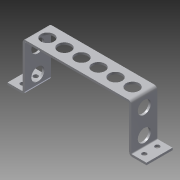
# Autodesk Inventor part: M - Lower Rail Connector Bracket 1
Saved by Autodesk Inventor 2013 (Build 170138000, 138)
## iProperties
Created: 2013-02-17
Part Number: M - Lower Rail Connector Bracket 1
Material: Aluminum 6061
Document SubType Name: Sheet Metal
Designer: Moses
Density: 2.71 g/cm^3
Sheet Metal Rule: Default
Mass: 82.9622 g
Surface Area: 238.016 cm^2
Volume: 30.6134 cm^3
Author: Moses
Autodesk Inventor part; units mm, degrees
ref_plane "YZ Plane" through (0, 0, 0) normal (1, 0, 0) x (0, 1, 0)
ref_plane "XZ Plane" through (0, 0, 0) normal (0, 1, 0) x (-1, 0, 0)
ref_plane "XY Plane" through (0, 0, 0) normal (0, 0, 1) x (1, 0, 0)
sketch "Sketch1" plane through (0, 0, 0) normal (0, 1, 0) x (-1, 0, 0)
  line L0 (0, 0) -> (0, 38.1)
  line L1 (0, 38.1) -> (25.4, 38.1)
  line L2 (25.4, 38.1) -> (25.4, 0)
  line L3 (25.4, 0) -> (0, 0)
  line L4 (12.7, 38.1) -> (12.7, 0) construction
  circle A0 centre (12.7, 28.575) radius 3.3782
  circle A1 centre (12.7, 9.525) radius 3.3782
  dimension "d0" = 38.1
  dimension "d1" = 25.4
  dimension "d2" = 6.7564
  dimension "d3" = 19.05
  dimension "d4" = 9.525
  measures "d0" distance of L0.start L0.end
  measures "d1" distance of L0.end L1.end
  measures "d2" diameter of A0
  measures "d3" distance of A1.centre A0.centre
  measures "d4" distance from line of L1 A0.centre
extrude "Plate1" add sketch "Sketch1" along normal blind 3.175
sketch "Sketch2" plane through (-22.225, 0, 38.1) normal (-1, 0, 0) x (0, -1, 0)
  line L0 (0, -38.1) -> (0, 0)
  line L1 (0, 0) -> (-69.85, 0)
  line L2 (-69.85, 0) -> (-69.85, -38.1)
  line L3 (-69.85, -38.1) -> (0, -38.1)
  constraints: 6 end point, 1 horizontal, 1 perpendicular, 1 vertical
edge flange "Flange1" height 69.85 angle 90 thickness 3.175 bend radius 1.27 thickness toward (-1, 0, 0) relief tear relief width 3.175 relief depth 1.5875 edges at (-25.4, 3.175, 19.05) wall of the first edge with corners at (-22.225, 0, 0) (-22.225, 0, 38.1) (-22.225, 69.85, 38.1) (-22.225, 69.85, 0)
bend "Bend1"
corner "Corner1"
sketch "Sketch3" plane through (-22.225, 66.675, 0) normal (0, 1, 0) x (-1, 0, 0)
  line L0 (0, 38.1) -> (0, 0)
  line L1 (0, 0) -> (158.75, 0)
  line L2 (158.75, 0) -> (158.75, 38.1)
  line L3 (158.75, 38.1) -> (0, 38.1)
  constraints: 6 end point, 1 horizontal, 1 perpendicular, 1 vertical
edge flange "Flange2" height 158.75 angle 90 thickness 3.175 bend radius 1.27 thickness toward (0, 1, 0) relief tear relief width 3.175 relief depth 1.5875 edges at (-25.4, 69.85, 19.05) wall of the first edge with corners at (-22.225, 66.675, 38.1) (-22.225, 66.675, 0) (-180.975, 66.675, 0) (-180.975, 66.675, 38.1)
bend "Bend2"
corner "Corner2"
sketch "Sketch4" plane through (-177.8, 69.85, 0) normal (-1, 0, 0) x (0, -1, 0)
  line L0 (0, 38.1) -> (0, 0)
  line L1 (0, 0) -> (69.85, 0)
  line L2 (69.85, 0) -> (69.85, 38.1)
  line L3 (69.85, 38.1) -> (0, 38.1)
  constraints: 6 end point, 1 horizontal, 1 perpendicular, 1 vertical
edge flange "Flange3" height 69.85 angle 90 thickness 3.175 bend radius 1.27 thickness toward (-1, 0, 0) relief tear relief width 3.175 relief depth 1.5875 edges at (-180.975, 66.675, 19.05) wall of the first edge with corners at (-177.8, 69.85, 38.1) (-177.8, 69.85, 0) (-177.8, 0, 0) (-177.8, 0, 38.1)
bend "Bend3"
corner "Corner3"
sketch "Sketch5" plane through (-177.8, 3.175, 38.1) normal (0, -1, 0) x (1, 0, 0)
  line L0 (0, -38.1) -> (0, 0)
  line L1 (0, 0) -> (-25.4, 0)
  line L2 (-25.4, 0) -> (-25.4, -38.1)
  line L3 (-25.4, -38.1) -> (0, -38.1)
  constraints: 6 end point, 1 horizontal, 1 perpendicular, 1 vertical
edge flange "Flange4" height 25.4 angle 90 thickness 3.175 bend radius 1.27 thickness toward (0, -1, 0) relief tear relief width 3.175 relief depth 1.5875 edges at (-180.975, 0, 19.05) wall of the first edge with corners at (-177.8, 3.175, 0) (-177.8, 3.175, 38.1) (-203.2, 3.175, 38.1) (-203.2, 3.175, 0)
bend "Bend4"
corner "Corner4"
sketch "Sketch6" plane through (-203.2, 0, 0) normal (0, -1, 0) x (1, 0, 0)
  line L0 (0, 38.1) -> (20.955, 38.1) projected
  line L1 (0, 0) -> (0, 38.1) projected
  line L2 (20.955, 0) -> (0, 0) projected
  line L3 (12.7, 38.1) -> (12.7, 0) construction
  circle A0 centre (12.7, 28.575) radius 3.3782
  circle A1 centre (12.7, 9.525) radius 3.3782
  point P0 (203.2, 0)
  dimension "d46" = 12.7
  dimension "d47" = 6.7564
  dimension "d48" = 19.05
  dimension "d49" = 9.525
  constraints: 4 point on line, 2 centre point, 2 end point, 1 equal radius, 1 perpendicular
  measures "d46" distance between parallel lines of L3 L1
  measures "d47" diameter of A0
  measures "d48" distance of A1.centre A0.centre
  measures "d49" distance from line of L0 A0.centre
extrude "Cut1" cut sketch "Sketch6" against normal blind 3.175
sketch "Sketch7" plane through (-26.67, 69.85, 38.1) normal (0, 1, 0) x (1, 0, 0)
  line L0 (-149.86, 38.1) -> (-149.86, 0) projected
  line L1 (0, 0) -> (0, 38.1) projected
  circle A0 centre (-137.16, 19.05) radius 9.525
  line L2 (-149.86, 19.05) -> (0, 19.05) construction
  circle A1 centre (-112.268, 19.05) radius 9.525
  circle A2 centre (-87.376, 19.05) radius 9.525
  circle A3 centre (-62.484, 19.05) radius 9.525
  circle A4 centre (-37.592, 19.05) radius 9.525
  circle A5 centre (-12.7, 19.05) radius 9.525
  point P0 (26.67, 38.1)
  dimension "d52" = 149.86
  dimension "d53" = 12.7
  dimension "d56" = 24.892
  dimension "d61" = 19.05
  constraints: 6 centre point, 2 end point, 2 midpoint, 1 horizontal, 1 point on line, 10 other
  measures "d52" distance of L0.start L1.end
  measures "d53" distance from line of A0.centre L0
  measures "d56" distance of A0.centre A1.centre
  measures "d61" diameter of A0
extrude "Cut2" cut sketch "Sketch7" against normal blind 3.175
sketch "Sketch8" plane through (-180.975, 65.405, 0) normal (-1, 0, 0) x (0, 0, 1)
  line L0 (0, -60.96) -> (38.1, -60.96) projected
  line L1 (38.1, 0) -> (0, 0) projected
  line L2 (19.05, 0) -> (19.05, -60.96) construction
  circle A0 centre (19.05, -12.7) radius 9.525
  circle A1 centre (19.05, -48.26) radius 9.525
  point P0 (0, -65.405)
  dimension "d64" = 19.05
  dimension "d66" = 12.7
  dimension "d67" = 12.7
  constraints: 2 centre point, 2 end point, 2 midpoint, 2 point on line, 1 equal radius
  measures "d64" diameter of A0
  measures "d66" distance from line of L1 A0.centre
  measures "d67" distance from line of L0 A1.centre
extrude "Cut3" cut sketch "Sketch8" against normal blind 5080
equation "\"d50\" = Thickness"
equation "\"d56\" = -0.4 * d53 + 0.2 * d52"
equation "\"d62\" = Thickness"
equation "\"d6\" = BendReliefWidth"
equation "\"d7\" = BendReliefDepth"
equation "\"d8\" = MinimumRemnant"
equation "\"d9\" = BendRadius"
equation "\"d13\" = CornerReliefSize"
equation "\"d14\" = GapSize"
equation "\"d15\" = JacobiRadiusSize"
equation "\"d16\" = BendReliefWidth"
equation "\"d17\" = BendReliefDepth"
equation "\"d18\" = MinimumRemnant"
equation "\"d19\" = BendRadius"
equation "\"d23\" = CornerReliefSize"
equation "\"d24\" = GapSize"
equation "\"d25\" = JacobiRadiusSize"
equation "\"d26\" = BendReliefWidth"
equation "\"d27\" = BendReliefDepth"
equation "\"d28\" = MinimumRemnant"
equation "\"d29\" = BendRadius"
equation "\"d33\" = CornerReliefSize"
equation "\"d34\" = GapSize"
equation "\"d35\" = JacobiRadiusSize"
equation "\"d36\" = BendReliefWidth"
equation "\"d37\" = BendReliefDepth"
equation "\"d38\" = MinimumRemnant"
equation "\"d39\" = BendRadius"
equation "\"d43\" = CornerReliefSize"
equation "\"d44\" = GapSize"
equation "\"d45\" = JacobiRadiusSize"
equation "\"BendRadius\" = Thickness"
equation "\"BendReliefWidth\" = Thickness"
equation "\"BendReliefDepth\" = 0.5 * Thickness"
equation "\"CornerReliefSize\" = 4 * Thickness"
equation "\"MinimumRemnant\" = 2 * Thickness"
equation "\"TransitionRadius\" = BendRadius"
equation "\"JacobiRadiusSize\" = BendRadius"
equation "\"GapSize\" = Thickness"
equation "\"d5\" = BendRadius"
equation "\"Thickness\" = 3.175"
body "Solid1"
